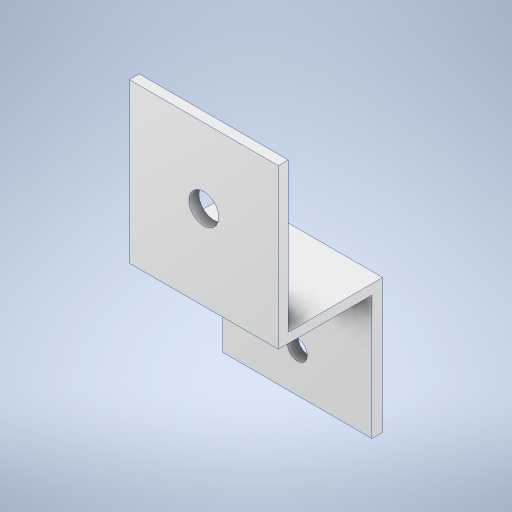
# Autodesk Inventor part: transversal-2l-stabilizer
Saved by Autodesk Inventor 2024 (Build 280153000, 153)
## iProperties
Created: 2025-12-12
Part Number: transversal-2l-stabilizer
Material: Aluminum 6061
Document SubType Name: Modeling
Designer: schar
Density: 2.7 g/cm^3
Appearance: Aluminum - Flat
Author: schar
Autodesk Inventor part; units mm, degrees
ref_plane "YZ Plane" through (0, 0, 0) normal (1, 0, 0) x (0, 1, 0)
ref_plane "XZ Plane" through (0, 0, 0) normal (0, 1, 0) x (-1, 0, 0)
ref_plane "XY Plane" through (0, 0, 0) normal (0, 0, 1) x (1, 0, 0)
sketch "Sketch1" plane through (0, 0, 0) normal (1, 0, 0) x (0, 1, 0)
  line L0 (0, 0) -> (-2, 0)
  line L1 (-2, 0) -> (-2, -19)
  line L2 (-2, -19) -> (0, -19)
  line L3 (0, -19) -> (0, 0)
  line L4 (0, 0) -> (30, 0)
  line L5 (30, 0) -> (30, 2)
  line L6 (30, 2) -> (0, 2)
  line L7 (0, 2) -> (0, 0)
  line L8 (-2, -19) -> (-32, -19)
  line L9 (-32, -19) -> (-32, -16.849)
  line L10 (-32, -16.849) -> (-2, -16.849)
  line L11 (-2, -16.849) -> (-2, -19)
  line L12 (0, 0) -> (-2, 0)
  line L13 (-2, 0) -> (-2, 2)
  line L14 (-2, 2) -> (0, 2)
  line L15 (0, 2) -> (0, 0)
  point P0 (-2, -16.849)
  dimension "d0" = 2
  dimension "d1" = 19
  dimension "d2" = 30
  dimension "d3" = 2
  dimension "d4" = 30
  constraints: 32 end point, 8 parallel, 4 horizontal, 4 perpendicular
  measures "d0" distance of L2.end L1.end
  measures "d1" distance of L1.end L0.end
  measures "d2" distance of L6.end L5.end
  measures "d3" distance of L5.end L4.end
  measures "d4" distance of L9.end L10.end
extrude "Extrusion1" add sketch "Sketch1" along normal blind 30
sketch "Sketch2" plane through (0, -2, 2) normal (0, 0, 1) x (1, 0, 0)
  line L0 (0, 0) -> (30, 0) projected
  line L1 (0, 0) -> (15, 0)
  line L2 (15, 0) -> (15, 17)
  circle A0 centre (15, 17) radius 3
  point P0 (0, 2)
  dimension "d7" = 17
  dimension "d8" = 6
  constraints: 4 end point, 1 centre point, 1 coincident, 1 horizontal, 1 perpendicular
  measures "d7" distance of L1.end L2.end
  measures "d8" diameter of A0
hole "Hole1" at (15, 15, 2) direction (0, 0, -1) diameter 6 end through all
sketch "Sketch4" plane through (0, -32, -19) normal (0, 0, -1) x (-1, 0, 0)
  line L0 (0, 32) -> (-15, 32)
  line L1 (0, 32) -> (-30, 32) projected
  line L2 (-15, 32) -> (-15, 13)
  dimension "d25" = 19
  constraints: 4 end point, 1 midpoint, 1 perpendicular
  measures "d25" distance of L0.end L2.end
hole "Hole3" at (15, -19, -19) direction (0, 0, 1) diameter 4 end through all
sketch "Sketch5" plane through (0, -32, -19) normal (0, -1, 0) x (1, 0, 0)
  line L0 (0, 0) -> (30, 0) projected
  line L1 (0, 2.151) -> (30, 2.151) projected
  line L2 (30, 0) -> (0, 0)
  line L3 (0, 0) -> (0, 2.151)
  line L4 (0, 2.151) -> (30, 2.151)
  line L5 (30, 2.151) -> (30, 0)
  point P0 (0, 19)
  constraints: 8 end point, 2 parallel, 1 horizontal, 1 perpendicular
extrude "Extrusion2" cut sketch "Sketch5" against normal blind 5
thread "Thread1" size "M4x0.7" class "6H" standard "ANSI Metric M Profile" length 70
body "Solid1"
